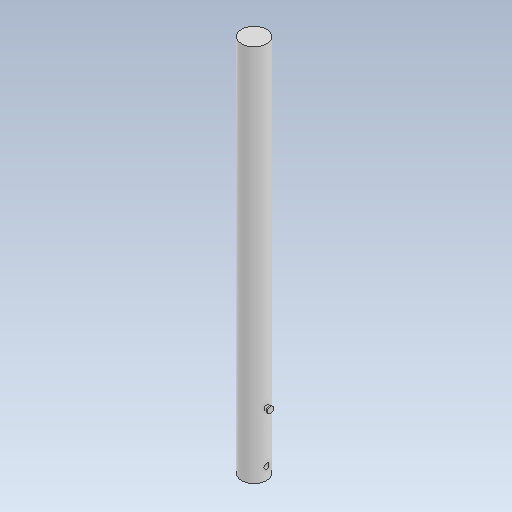
# Autodesk Inventor part: trail 9
Saved by Autodesk Inventor 2020.2 (Build 242310000, 310)
## iProperties
Created: 2020-02-17
Part Number: trail 9
Material: Generic
Document SubType Name: Modeling
Designer: lenovo
Density: 1 g/cm^3
Appearance: Default
Mass: 94.0427 g
Surface Area: 197.572 cm^2
Volume: 94.0427 cm^3
Author: lenovo
Autodesk Inventor part; units mm, degrees
ref_plane "YZ Plane" through (0, 0, 0) normal (1, 0, 0) x (0, 1, 0)
ref_plane "XZ Plane" through (0, 0, 0) normal (0, 1, 0) x (-1, 0, 0)
ref_plane "XY Plane" through (0, 0, 0) normal (0, 0, 1) x (1, 0, 0)
sketch "Sketch1" plane through (0, 0, 0) normal (0, 1, 0) x (-1, 0, 0)
  circle A0 centre (0, 0) radius 10
  dimension "d0" = 20
  constraints: 1 centre point, 1 coincident
  measures "d0" diameter of A0
extrude "Extrusion1" add sketch "Sketch1" along normal blind 300
sketch "Sketch2" plane through (0, 0, 0) normal (1, 0, 0) x (0, 1, 0)
  circle A0 centre (10, 0) radius 2
  circle A1 centre (50, 0) radius 2
  point P0 (0, 0)
  dimension "d3" = 4
  dimension "d4" = 4
  constraints: 2 centre point
  measures "d3" diameter of A0
  measures "d4" diameter of A1
extrude "Extrusion2" cut sketch "Sketch2" along normal mid plane 21 contours A0
sketch "Sketch3" plane through (0, 0, 0) normal (1, 0, 0) x (0, 1, 0)
  circle A0 centre (50, 0) radius 2
  point P0 (0, 0)
  dimension "d7" = 4
  constraints: 1 centre point
  measures "d7" diameter of A0
extrude "Extrusion3" add sketch "Sketch3" along normal blind 12
sketch "Sketch4" plane through (12, 50, 0) normal (1, 0, 0) x (0, 0, -1)
  circle A0 centre (0, 0) radius 2 projected
  circle A1 centre (0, 0) radius 2.5
  point P0 (0, -50)
  dimension "d10" = 5
  constraints: 1 centre point, 1 coincident
  measures "d10" diameter of A1
extrude "Extrusion4" add sketch "Sketch4" along normal blind 1 contours A0 | A1
body "Solid1"
